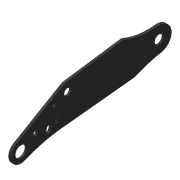
# Autodesk Inventor part: UPPER_LEG_OUTER_FRAME
Saved by Autodesk Inventor 2019.4 (Build 234330000, 330)
## iProperties
Created: 2019-11-12
Part Number: UPPER_LEG_OUTER_FRAME
Material: 一般
Document SubType Name: Modeling
Designer: y6tada
Density: 1 g/cm^3
Appearance: Black 80
Author: y6tada
Autodesk Inventor part; units mm, degrees
ref_plane "YZ Plane" through (0, 0, 0) normal (1, 0, 0) x (0, 1, 0)
ref_plane "XZ Plane" through (0, 0, 0) normal (0, 1, 0) x (-1, 0, 0)
ref_plane "XY Plane" through (0, 0, 0) normal (0, 0, 1) x (1, 0, 0)
sketch "スケッチ1" plane through (0, 0, 0) normal (1, 0, 0) x (0, 1, 0)
  line L0 (0, 0) -> (-25, 122.4745) construction
  line L1 (0, 189.3993) -> (0, 0) construction
  line L2 (7.4223, 85.1346) -> (-15.7417, 127.5327)
  arc A0 (-15.7417, 127.5327) -> (-34.3869, 117.6589) centre (-25, 122.4745) ccw
  arc A1 (8.3366, 82.3958) -> (7.4223, 85.1346) centre (0.2614, 81.2223) ccw
  arc A2 (-16.6192, 127.0533) -> (-30.6712, 114.7908) centre (-25, 122.4745) ccw construction
  circle A3 centre (0.2614, 81.2223) radius 7.16 construction
  line L3 (7.347, 82.252) -> (18.9014, 2.7469) construction
  line L4 (6.5448, 84.6552) -> (-16.6192, 127.0533) construction
  line L5 (-30.6712, 114.7908) -> (-18.354, 105.6997) construction
  line L6 (-16.6291, 102.1772) -> (-19.0944, 0.4628) construction
  arc A4 (-16.6291, 102.1772) -> (-18.354, 105.6997) centre (-20.8779, 102.2802) ccw construction
  circle A5 centre (-20.8779, 102.2802) radius 4 construction
  arc A6 (-21.5454, 102.6936) -> (-20.1769, 101.9265) centre (-16.4772, 110.131) ccw construction
  arc A7 (-20.3909, 104.3877) -> (-20.2189, 104.2741) centre (-16.4772, 110.131) ccw
  arc A8 (-22.6998, 100.9996) -> (-21.0196, 100.0578) centre (-16.4772, 110.131) ccw
  arc A9 (-21.0196, 100.0578) -> (-19.3342, 103.7953) centre (-20.1769, 101.9265) ccw
  arc A10 (-20.3909, 104.3877) -> (-22.6998, 100.9996) centre (-21.5454, 102.6936) ccw
  line L7 (-20.1769, 101.9265) -> (-16.4772, 110.131) construction
  line L8 (-16.4772, 110.131) -> (-21.5454, 102.6936) construction
  circle A11 centre (-16.4772, 110.131) radius 2.05
  line L9 (-25, 122.4745) -> (-16.4772, 110.131) construction
  arc A12 (15.1465, 30.5862) -> (10.9324, 1.2173) centre (69.7422, 7.7656) ccw
  arc A13 (-10.7575, -2.297) -> (10.9324, 1.2173) centre (0, 0) ccw
  arc A14 (-10.7575, -2.297) -> (-19.0681, 23.5944) centre (-143.6482, -30.673) ccw
  line L10 (15.4813, 33.2335) -> (8.3366, 82.3958)
  line L11 (-18.1011, 82.7172) -> (-19.4827, 25.7123)
  line L12 (5.3923, 89.8056) -> (-23.9461, 86.722) construction
  line L13 (13.2872, 33.8242) -> (7.5904, 88.0256) construction
  line L14 (-16.4772, 110.131) -> (-20.8779, 102.2802) construction
  arc A15 (-19.5208, 103.8828) -> (-20.2189, 104.2741) centre (-20.8779, 102.2802) ccw
  arc A16 (-20.2189, 104.2741) -> (-19.5208, 103.8828) centre (-16.4772, 110.131) ccw construction
  arc A17 (-19.5208, 103.8828) -> (-19.3342, 103.7953) centre (-16.4772, 110.131) ccw
  arc A18 (-12.7543, 90.4805) -> (-9.3986, 91.4255) centre (-16.4772, 110.131) ccw construction
  line L15 (-9.3986, 91.4255) -> (-16.4772, 110.131) construction
  line L16 (-12.7543, 90.4805) -> (-16.4772, 110.131) construction
  arc A19 (-12.9498, 91.5122) -> (-9.7703, 92.4076) centre (-16.4772, 110.131) ccw
  arc A20 (-12.5589, 89.4489) -> (-9.027, 90.4435) centre (-16.4772, 110.131) ccw
  arc A21 (-9.027, 90.4435) -> (-9.7703, 92.4076) centre (-9.3986, 91.4255) ccw
  arc A22 (-12.9498, 91.5122) -> (-12.5589, 89.4489) centre (-12.7543, 90.4805) ccw
  line L17 (0, 0) -> (-9.0564, 86.1659) construction
  line L18 (17.4675, 35.8375) -> (13.9144, 27.8571) construction
  line L19 (-19.4021, 24.3553) -> (-21.3765, 28.7898) construction
  line L20 (-16.4772, 110.131) -> (-11.0559, 90.8798) construction
  arc A23 (-18.7518, 87.7462) -> (-7.9406, 89.3133) centre (-16.4772, 110.131) ccw construction
  arc A24 (-19.0944, 0.4628) -> (18.9014, 2.7469) centre (0, 0) ccw construction
  line L21 (-34.3869, 117.6589) -> (-19.4205, 88.4854)
  arc A25 (-18.1011, 82.7172) -> (-19.4205, 88.4854) centre (-30.0975, 83.008) ccw
  circle A26 centre (-20.8779, 102.2802) radius 5 construction
  arc A27 (15.1465, 30.5862) -> (15.4813, 33.2335) centre (10.5333, 32.5144) ccw
  arc A28 (-19.4827, 25.7123) -> (-19.0681, 23.5944) centre (-14.4842, 25.5912) ccw
  point P0 (10.0992, 80.235)
  point P1 (-17.9888, 87.3482)
  point P2 (15.6848, 31.8335)
  point P3 (-19.5097, 24.5971)
  point P4 (0, 0)
  dimension "d2" = 125
  dimension "d10" = 19.1
  dimension "d11" = 14.32
  dimension "d13" = 8
  dimension "d14" = 0.25
  dimension "d18" = 9
  dimension "d19" = 10
  dimension "d20" = 4.1
  dimension "d25" = 11
  dimension "d30" = 8
  dimension "d35" = 15
  dimension "d38" = 2.1
  dimension "d40" = 10
  dimension "d41" = 1.05
  dimension "d42" = 8
  dimension "d70" = 45
  dimension "d72" = 20
  dimension "d73" = 2.05
  dimension "d74" = 2.5
  dimension "d75" = 19.1
  dimension "d76" = 6
  dimension "d77" = 25
  dimension "d78" = 1
  dimension "d79" = 1
  dimension "d80" = 12
  dimension "d81" = 1
  dimension "d82" = 1
  dimension "d83" = 5
  constraints: 59 point on circle, 40 end point, 32 tangent, 29 centre point, 13 coincident, 11 point on line, 2 concentric, 2 parallel, 1 equal radius, 1 vertical, 7 other
  measures "d2" distance of L0.end L0.start
  measures "d10" diameter of A2
  measures "d11" diameter of A3
  measures "d13" diameter of A5
  measures "d14" radial gap between concentric circles of A5 A4
  measures "d18" radius of A6
  measures "d19" angle of L7 L8
  measures "d20" diameter of A11
  measures "d25" radius of A13
  measures "d30" distance from line of L13 A1.centre
  measures "d35" distance of L0.end L9.end
  measures "d38" radius of A15
  measures "d40" angle of L15 L16
  measures "d41" radius of A21
  measures "d42" distance from line of L12 A1.centre
  measures "d70" angle of L14 L20
  measures "d72" radius of A18
  measures "d73" radius of A9
  measures "d74" radial gap between concentric circles of A23 A18
  measures "d75" radius of A24
  measures "d76" angle of L1 L17
  measures "d77" distance from line of A0.centre L1
  measures "d78" distance between parallel lines of L10 L3
  measures "d79" radial gap between concentric circles of A0 A2
  measures "d80" radius of A25
  measures "d81" distance between parallel lines of L11 L6
  measures "d82" radial gap between concentric circles of A5 A26
  measures "d83" radius of A27
extrude "押し出し1" add sketch "スケッチ1" along normal blind 2
hole "穴1" at (0, 0, 0) direction (1, 0, 0) diameter 8 end through all counterbore diameter 9.3 counterbore depth 0.65
hole "穴2" at (0, 0.2614, 81.2223) direction (1, 0, 0) diameter 6 end through all counterbore diameter 7.3 counterbore depth 0.65
hole "穴3" at (0, -25, 122.4745) direction (1, 0, 0) diameter 10 end through all counterbore diameter 11.3 counterbore depth 0.65
